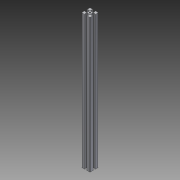
# Autodesk Inventor part: Rail_Misumi_HFS3-1515-240
Saved by Autodesk Inventor 2014 (Build 180170000, 170)
## iProperties
Created: 2014-01-09
Part Number: Rail_Misumi_HFS3-1515-240
Material: Aluminum 6061
Document SubType Name: Modeling
Designer: ThatOtherGuy
Density: 2.71 g/cm^3
Mass: 89.3382 g
Surface Area: 307.071 cm^2
Volume: 32.9661 cm^3
Appearance: Aluminum - Flat
Author: ThatOtherGuy
Autodesk Inventor part; units mm, degrees
ref_plane "YZ Plane" through (0, 0, 0) normal (1, 0, 0) x (0, 1, 0)
ref_plane "XZ Plane" through (0, 0, 0) normal (0, 1, 0) x (-1, 0, 0)
ref_plane "XY Plane" through (0, 0, 0) normal (0, 0, 1) x (1, 0, 0)
sketch "Sketch1" plane through (0, 0, 0) normal (0, 0, 1) x (1, 0, 0)
  line L0 (0, 0) -> (0, 5.8)
  line L1 (0, 5.8) -> (1.1, 5.8)
  line L2 (1.1, 5.8) -> (1.1, 4.65)
  line L3 (4.7, 5.8) -> (4.7, 9.2)
  line L4 (1.1, 10.35) -> (1.1, 9.2)
  line L5 (1.1, 9.2) -> (0, 9.2)
  line L6 (0, 9.2) -> (0, 15)
  line L7 (0, 15) -> (5.8, 15)
  line L8 (5.8, 15) -> (5.8, 13.9)
  line L9 (5.8, 13.9) -> (4.65, 13.9)
  line L10 (5.8, 10.3) -> (9.2, 10.3)
  line L11 (10.35, 13.9) -> (9.2, 13.9)
  line L12 (9.2, 13.9) -> (9.2, 15)
  line L13 (9.2, 15) -> (15, 15)
  line L14 (15, 15) -> (15, 9.2)
  line L15 (15, 9.2) -> (13.9, 9.2)
  line L16 (13.9, 9.2) -> (13.9, 10.35)
  line L17 (10.3, 9.2) -> (10.3, 5.8)
  line L18 (13.9, 4.65) -> (13.9, 5.8)
  line L19 (13.9, 5.8) -> (15, 5.8)
  line L20 (15, 5.8) -> (15, 0)
  line L21 (15, 0) -> (9.2, 0)
  line L22 (9.2, 0) -> (9.2, 1.1)
  line L23 (9.2, 1.1) -> (10.35, 1.1)
  line L24 (9.2, 4.7) -> (5.8, 4.7)
  line L25 (4.65, 1.1) -> (5.8, 1.1)
  line L26 (5.8, 1.1) -> (5.8, 0)
  line L27 (5.8, 0) -> (0, 0)
  circle A0 centre (7.5, 7.5) radius 1.25
  line L28 (1.1, 10.35) -> (3.7, 10.35)
  line L29 (3.7, 10.35) -> (4.7, 9.2)
  line L30 (4.7, 5.8) -> (3.7, 4.65)
  line L31 (3.7, 4.65) -> (1.1, 4.65)
  line L32 (4.65, 13.9) -> (4.65, 11.3)
  line L33 (4.65, 11.3) -> (5.8, 10.3)
  line L34 (9.2, 10.3) -> (10.35, 11.3)
  line L35 (10.35, 11.3) -> (10.35, 13.9)
  line L36 (13.9, 10.35) -> (11.3, 10.35)
  line L37 (11.3, 10.35) -> (10.3, 9.2)
  line L38 (10.3, 5.8) -> (11.3, 4.65)
  line L39 (11.3, 4.65) -> (13.9, 4.65)
  line L40 (10.35, 1.1) -> (10.35, 3.7)
  line L41 (10.35, 3.7) -> (9.2, 4.7)
  line L42 (5.8, 4.7) -> (4.65, 3.7)
  line L43 (4.65, 3.7) -> (4.65, 1.1)
  arc A1 (1, 15) -> (0, 14) centre (1, 14) ccw
  arc A2 (15, 14) -> (14, 15) centre (14, 14) ccw
  arc A3 (14, 0) -> (15, 1) centre (14, 1) ccw
  arc A4 (0, 1) -> (1, 0) centre (1, 1) ccw
  dimension "d6" = 15
  dimension "d7" = 1.1
  dimension "d8" = 5.7
  dimension "d9" = 3.4
  dimension "d10" = 2.5
  dimension "d13" = 7.5
  dimension "d14" = 7.5
  dimension "d18" = 15
  dimension "d19" = 3.6
  dimension "d20" = 1
  dimension "d21" = 3.4
  dimension "d22" = 1
  constraints: 88 end point, 38 equal length, 14 horizontal, 14 vertical, 8 point on circle, 8 point on line, 8 tangent, 6 parallel, 5 centre point, 3 equal radius, 3 perpendicular, 2 horizontal alignment, 2 vertical alignment
  measures "d6" distance between parallel lines of L20 L0
  measures "d7" distance of L4.end L5.end
  measures "d8" distance of L2.end L4.start
  measures "d9" distance between parallel lines of L5 L1
  measures "d10" diameter of A0
  measures "d13" horizontal distance of L0.start A0.centre
  measures "d14" horizontal distance of L0.start A0.centre
  measures "d18" distance of L20.end L13.end
  measures "d19" distance between parallel lines of L2 L3
  measures "d20" horizontal distance of L3.end L28.end
  measures "d21" distance of L3.start L3.end
  measures "d22" radius of A1
extrude "Extrusion1" add sketch "Sketch1" along normal blind 240 contours L0 L1 L2 L31 L30 L3 L29 L28 L4 L5 L6 A1 L7 L8 L9 L32 L33 L10 L34 L35 L11 L12 L13 A2 L14 L15 L16 L36 L37 L17 L38 L39 L18 L19 L20 A3 L21 L22 L23 L40 L41 L24 L42 L43 L25 L26 L27 A4
equation "\"d13\" = 0.5 * d6"
equation "\"d14\" = 0.5 * d6"
equation "\"d18\" = d6"
equation "\"d21\" = d9"
body "Solid1"
